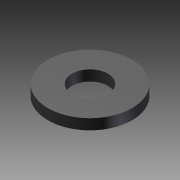
# Autodesk Inventor part: PACK-PWFN3
Saved by Autodesk Inventor 2011 SP1 (Build 150282100, 282)
## iProperties
Created: 2016-04-08
Part Number: PACK-PWFN3
Catalog Web Link: www.cadenas.de
Description: PACK-PWFN, PACK-SPWFN-Washers for Slotted Holes
Vendor: MISUMI
Document SubType Name: Modeling
Designer: psAdmin
Manufacturer: MISUMI
Mass: 0.0411863 g
Surface Area: 1.18187 cm^2
Volume: 0.0411863 cm^3
Density: 1 g/cm^3
Category: PARTsolutions
Company: MISUMI
Title: PACK-PWFN3
Author: Cadenas PARTsolutions
Comments: Washers for Slotted Holes
PSOL_IDENT_0: {$CADENAS_DATA\23d-libs\misumi\metric\27_screws_nuts\pack_pwfn.prj},180 {VTYP=3D},{NB=PACK-PWFN3},{L
PSOL_IDENT_1: INA=PACK-PWFN3},{NN=PACK-PWFN, PACK-SPWFN},{DATE=29.07.2015 04:50:06},{GEOMDATE=31.05.2011 01:58:00}
PSOL_IDENT_2: ,{VERSION=},{LINEID=10},{LINESUBID=-1},{WBVAR=MAT}  {NB=PACK-PWFN3},{LINA=PACK-PWFN3},{KT=DUMMY},{PN=
PSOL_IDENT_3: PACK-PWFN3},{TYPE=PACK-PWFN},{MAT=},{ST=Trivalent Chromate},{NO=3},{DD=3.4},{DD1=3.4},{DD2=3.3},{D=8
PSOL_IDENT_4: },{D1=8},{D2=8},{TT=1.0},{TT1=1.0},{TT2=1.0},{PNO=50}
NN: PACK-PWFN, PACK-SPWFN
NT: Washers for Slotted Holes
NB: PACK-PWFN3
NBSYN: $PN.
LINA: PACK-PWFN3
PN: PACK-PWFN3
MAT: SPCC
ST: Trivalent Chromate
NO: 3
DD: 3.4
D: 8
TT: 1.0
PNO: 50
SUPPLIER: MISUMI
ARTICLENO: PACK-PWFN3
BOMINFO: PACK-PWFN3
CREATOR: CADENAS GmbH
Autodesk Inventor part; units mm, degrees
sketch "Sketch_1" plane through (0, 0, 0) normal (1, 0, 0) x (0, 1, 0)
  line L0 (0, -1) -> (0, 0)
  line L1 (4, 0) -> (1.7, 0)
  line L2 (1.7, 0) -> (1.7, -1)
  line L3 (1.7, -1) -> (4, -1)
  line L4 (4, -1) -> (4, 0)
  constraints: 10 end point
revolve "Revolution1" add sketch "Sketch_1" angle 360 about axis through (0, 0, -1) along (0, 0, -1)
ref_plane "C1_XY" through (0, 0, 0) normal (0, 0, -1) x (1, 0, 0)
ref_plane "C1_YZ" through (0, 0, 0) normal (1, 0, 0) x (0, -1, 0)
ref_plane "C1_ZX" through (0, 0, 0) normal (0, -1, 0) x (0, 0, -1)
body "Solid1"
